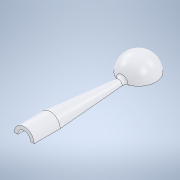
# Autodesk Inventor part: markerWithRodEnd
Saved by Autodesk Inventor 2022 (Build 260153000, 153)
## iProperties
Created: 2021-09-13
Part Number: markerWithRodEnd
Material: ABS Plastic
Document SubType Name: Modeling
Designer: tecware
Density: 1.06 g/cm^3
Appearance: Aluminum - Polished
Author: tecware
## iProperties of the stored document markerWithRodEnd_3DPrint.ipt
Created: 2021-09-13
Part Number: markerWithRodEnd_3DPrint
Material: Generic
Document SubType Name: Modeling
Designer: tecware
Density: 1 g/cm^3
Appearance: Default
Author: tecware
Autodesk Inventor part; units mm, degrees
ref_plane "YZ Plane" through (0, 0, 0) normal (1, 0, 0) x (0, 1, 0)
ref_plane "XZ Plane" through (0, 0, 0) normal (0, 1, 0) x (-1, 0, 0)
sketch "Sketch1" plane through (0, 0, 0) normal (0, 1, 0) x (-1, 0, 0)
  line L0 (0, 0) -> (-3.7, 0)
  line L1 (-3.7, 0) -> (-5.7, 0)
  line L2 (0, 0) -> (0, -40.75)
  line L3 (0, -40.75) -> (0, -50.75)
  circle A0 centre (0, -50.75) radius 10
  line L4 (-1.5, -40.8631) -> (0, -40.8631)
  line L5 (0, -40.8631) -> (0, -40.75)
  line L6 (-1.5, -40.75) -> (-1.5, -40.8631)
  line L7 (-1.5, -40.8631) -> (-3.7, 0)
  line L8 (0, -40.75) -> (-1.5, -40.75)
  line L9 (-1.5, -40.75) -> (-2, -40.75)
  line L10 (-2, -40.75) -> (-2, -40.952)
  line L11 (-2, -40.952) -> (-5.7, 0)
  line L12 (0, -50.75) -> (0, -60.75)
  circle A1 centre (0, -50.75) radius 9.2
  line L13 (-1.5, -40.8631) -> (-1.4568, -41.6661)
  line L14 (-3.7, 0) -> (-3.7, 15)
  line L15 (-3.7, 15) -> (-0.2, 15)
  line L16 (-5.7, 0) -> (-5.7, 15)
  line L17 (-5.7, 15) -> (-3.7, 15)
  point P0 (0, -59.95)
  dimension "d7" = 18.4
  dimension "d0" = 3.7
  dimension "d1" = 2
  dimension "d2" = 40.75
  dimension "d4" = 10
  dimension "d6" = 0.5
  dimension "d9" = 15
  constraints: 36 end point, 5 perpendicular, 4 point on circle, 4 vertical, 3 point on line, 2 coincident, 2 horizontal, 1 centre point, 1 parallel, 1 tangent, 3 other
  measures "d0" distance of L0.start L0.end
  measures "d1" distance of L0.end L1.end
  measures "d2" distance of L0.start L2.end
  measures "d4" distance of L2.end L3.end
  measures "d6" distance of L6.start L9.end
  measures "d9" distance of L0.end L14.end
revolve "Revolution1" add sketch "Sketch1" angle 180 about axis through (0, 0, 0) along (0, 0, 1) contours L7 L9 L10 L11 L1 | L1 L16 L17 L14 | L7 A0 L10 L9 | L13 A1 L12 A0
ref_plane "Work Plane1" through (3.7, 0, 0) normal (0, 0, 1) x (1, 0, 0)
sketch "Sketch2" plane through (3.7, 0, 0) normal (0, 0, 1) x (1, 0, 0)
  circle A0 centre (-3.7, 0) radius 3.7
  circle A1 centre (-3.7, 0) radius 2.2
  line L0 (2, 0) -> (-1.7, 0) projected
  line L1 (0, 0) -> (-7.4, 0)
  point P0 (-5.9, 0)
  point P1 (-1.5, 0)
  dimension "d13" = 4.4
  dimension "d14" = 7.4
  constraints: 2 centre point, 2 coincident, 2 end point, 2 point on circle, 1 collinear, 1 point on line
  measures "d13" diameter of A1
  measures "d14" diameter of A0
extrude "Rod Stopper" add sketch "Sketch2" against normal blind 2 contours L0 A1 L1 A0 picked at (-6.8429, 0.4707)
fillet "Fillet1" radius 2 1 edges at (0, 2, -40.952)
body "Solid1"
